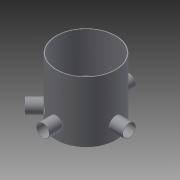
# Autodesk Inventor part: Vacuum Cylinder
Saved by Autodesk Inventor 2014 (Build 180170000, 170)
## iProperties
Created: 2014-05-19
Part Number: Vacuum Cylinder
Material: Generic
Document SubType Name: Modeling
Designer: ijs09
Density: 1 g/cm^3
Appearance: Default
Author: ijs09
Autodesk Inventor part; units mm, degrees
ref_plane "XY Plane" through (0, 0, 0) normal (0, 0, 1) x (1, 0, 0)
sketch "Sketch1" plane through (0, 0, 0) normal (0, 0, 1) x (1, 0, 0)
  circle A0 centre (0, 0) radius 98.552
  circle A1 centre (0, 0) radius 101.6
  dimension "d0" = 197.104
  dimension "d1" = 203.2
  constraints: 2 centre point, 2 coincident
  measures "d0" diameter of A0
  measures "d1" diameter of A1
extrude "Extrusion1" add sketch "Sketch1" along normal blind 205.64
ref_plane "Work Plane1" through (0, -101.6, 0) normal (0, 1, 0) x (-1, 0, 0)
ref_plane "Work Plane2" through (0, 101.6, 0) normal (0, 1, 0) x (-1, 0, 0)
ref_plane "Work Plane3" through (-101.6, 0, 0) normal (1, 0, 0) x (0, 1, 0)
ref_plane "Work Plane4" through (101.6, 0, 0) normal (1, 0, 0) x (0, 1, 0)
sketch "Sketch2" plane through (0, -101.6, 0) normal (0, 1, 0) x (-1, 0, 0)
  circle A0 centre (0, 50) radius 22.25
  line L0 (-101.6, 0) -> (101.6, 0) projected
  point P0 (0, 0)
  dimension "d4" = 44.5
  dimension "d5" = 50
  constraints: 1 centre point
  measures "d4" diameter of A0
  measures "d5" distance from line of A0.centre L0
extrude "Extrusion2" add sketch "Sketch2" against normal blind 44.7
sketch "Sketch3" plane through (0, -101.6, 0) normal (0, 1, 0) x (-1, 0, 0)
  circle A0 centre (0, 50) radius 19.05
  point P0 (0, 0)
  dimension "d8" = 38.1
  constraints: 1 centre point
  measures "d8" diameter of A0
extrude "Extrusion3" add sketch "Sketch3" along normal up to next
sketch "Sketch4" plane through (101.6, 0, 0) normal (1, 0, 0) x (0, 1, 0)
  circle A0 centre (0, 50) radius 22.25
  line L0 (-101.6, 0) -> (101.6, 0) projected
  point P0 (0, 0)
  dimension "d12" = 44.5
  dimension "d13" = 50
  constraints: 1 centre point
  measures "d12" diameter of A0
  measures "d13" distance from line of A0.centre L0
extrude "Extrusion4" add sketch "Sketch4" along normal blind 44.7
sketch "Sketch5" plane through (101.6, 0, 0) normal (1, 0, 0) x (0, 1, 0)
  circle A0 centre (0, 50) radius 19.05
  point P0 (0, 0)
  dimension "d16" = 38.1
  constraints: 1 centre point
  measures "d16" diameter of A0
extrude "Extrusion5" add sketch "Sketch5" against normal up to next
sketch "Sketch6" plane through (0, 101.6, 0) normal (0, 1, 0) x (-1, 0, 0)
  circle A0 centre (0, 50) radius 22.25
  line L0 (-101.6, 0) -> (101.6, 0) projected
  point P0 (0, 0)
  dimension "d22" = 44.5
  dimension "d23" = 50
  constraints: 1 centre point
  measures "d22" diameter of A0
  measures "d23" distance from line of A0.centre L0
extrude "Extrusion6" add sketch "Sketch6" along normal blind 44.7
sketch "Sketch7" plane through (0, 101.6, 0) normal (0, 1, 0) x (-1, 0, 0)
  circle A0 centre (0, 50) radius 19.05
  point P0 (0, 0)
  dimension "d26" = 38.1
  constraints: 1 centre point
  measures "d26" diameter of A0
extrude "Extrusion7" add sketch "Sketch7" against normal up to next
sketch "Sketch8" plane through (-101.6, 0, 0) normal (1, 0, 0) x (0, 1, 0)
  circle A0 centre (0, 50) radius 9.65
  line L0 (-101.6, 0) -> (101.6, 0) projected
  point P0 (0, 0)
  dimension "d32" = 19.3
  dimension "d33" = 50
  constraints: 1 centre point
  measures "d32" diameter of A0
  measures "d33" distance from line of A0.centre L0
extrude "Extrusion8" add sketch "Sketch8" against normal blind 15
sketch "Sketch9" plane through (-101.6, 0, 0) normal (1, 0, 0) x (0, 1, 0)
  circle A0 centre (0, 50) radius 9.65
  point P0 (0, 0)
  dimension "d36" = 19.3
  constraints: 1 centre point
  measures "d36" diameter of A0
extrude "Extrusion9" add sketch "Sketch9" along normal up to next
hole "Hole1" at (-116.6, 0, 50) direction (1, 0, 0) diameter 17.3 depth 100
hole "Hole2" at (146.3, 0, 50) direction (-1, 0, 0) diameter 42.5 depth 100
hole "Hole3" at (0, -146.3, 50) direction (0, 1, 0) diameter 42.5 end through all
ref_plane "Work Plane6" through (-71.842, 71.842, 0) normal (-0.7071068, 0.7071068, 0) x (-0.7071068, -0.7071068, 0)
ref_plane "Work Plane5" through (0, 0, 0) normal (-0.7071068, 0.7071068, 0) x (0, 0, 1)
sketch "Sketch10" plane through (-71.842, 71.842, 0) normal (-0.7071068, 0.7071068, 0) x (-0.7071068, -0.7071068, 0)
  circle A0 centre (0, 50) radius 22.25
  line L0 (-101.6, 0) -> (101.6, 0) projected
  point P0 (0, 0)
  dimension "d69" = 44.5
  dimension "d70" = 50
  constraints: 1 centre point
  measures "d69" diameter of A0
  measures "d70" distance from line of A0.centre L0
extrude "Extrusion10" add sketch "Sketch10" along normal blind 44.7
sketch "Sketch11" plane through (-71.842, 71.842, 0) normal (-0.7071068, 0.7071068, 0) x (-0.7071068, -0.7071068, 0)
  circle A0 centre (0, 50) radius 19.05
  point P0 (0, 0)
  dimension "d73" = 38.1
  constraints: 1 centre point
  measures "d73" diameter of A0
extrude "Extrusion11" add sketch "Sketch11" against normal up to next
hole "Hole4" at (-103.4497, 103.4497, 50) direction (0.7071068, -0.7071068, 0) diameter 42.5 depth 100
ref_plane "Work Plane8" through (-71.842, -71.842, 0) normal (0.7071068, 0.7071068, 0) x (-0.7071068, 0.7071068, 0)
ref_plane "Work Plane7" through (0, 0, 0) normal (0.7071068, 0.7071068, 0) x (0, 0, 1)
sketch "Sketch12" plane through (-71.842, -71.842, 0) normal (0.7071068, 0.7071068, 0) x (-0.7071068, 0.7071068, 0)
  circle A0 centre (0, 50) radius 22.25
  line L0 (-101.6, 0) -> (101.6, 0) projected
  point P0 (0, 0)
  dimension "d89" = 44.5
  dimension "d90" = 50
  constraints: 1 centre point
  measures "d89" diameter of A0
  measures "d90" distance from line of A0.centre L0
extrude "Extrusion12" add sketch "Sketch12" against normal blind 44.7
sketch "Sketch13" plane through (-71.842, -71.842, 0) normal (0.7071068, 0.7071068, 0) x (-0.7071068, 0.7071068, 0)
  circle A0 centre (0, 50) radius 19.05
  point P0 (0, 0)
  dimension "d93" = 38.1
  constraints: 1 centre point
  measures "d93" diameter of A0
extrude "Extrusion13" add sketch "Sketch13" along normal up to next
hole "Hole5" at (-103.4497, -103.4497, 50) direction (0.7071068, 0.7071068, 0) diameter 42.5 depth 100
equation "\"d12\" = d4"
equation "\"d13\" = d5"
equation "\"d16\" = d18"
equation "\"d22\" = d4"
equation "\"d23\" = d5"
equation "\"d26\" = d28"
equation "\"d33\" = d5"
equation "\"d69\" = d4"
equation "\"d70\" = d5"
equation "\"d73\" = d75"
equation "\"d89\" = d4"
equation "\"d90\" = d5"
equation "\"d93\" = d95"
equation "\"d18\" = 38.1"
equation "\"d28\" = 38.1"
equation "\"d75\" = 38.1"
equation "\"d95\" = 38.1"
body "Solid1"
